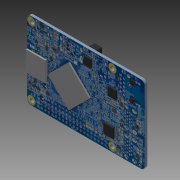
# Autodesk Inventor part: nanopi_m4_board
Saved by Autodesk Inventor 2013 SP2 (Build 170200200, 200)
## iProperties
Created: 2018-09-17
Part Number: nanopi_m4_board
Material: Generic
Document SubType Name: Modeling
Designer: alex
Density: 1 g/cm^3
Mass: 10.4345 g
Surface Area: 108.998 cm^2
Volume: 10.4345 cm^3
Author: alex
Autodesk Inventor part; units mm, degrees
ref_plane "YZ Plane" through (0, 0, 0) normal (1, 0, 0) x (0, 1, 0)
ref_plane "XZ Plane" through (0, 0, 0) normal (0, 1, 0) x (-1, 0, 0)
ref_plane "XY Plane" through (0, 0, 0) normal (0, 0, 1) x (1, 0, 0)
sketch "Sketch1" plane through (0, 0, 0) normal (0, 1, 0) x (-1, 0, 0)
  line L0 (0, 0) -> (-85, 0)
  line L1 (-85, 0) -> (-85, -56)
  line L2 (-85, -56) -> (0, -56)
  line L3 (0, -56) -> (0, 0)
  dimension "d0" = 85
  dimension "d1" = 56
  constraints: 8 end point, 2 parallel, 1 horizontal, 1 perpendicular
  measures "d0" distance of L2.end L1.end
  measures "d1" distance of L1.end L0.end
extrude "Extrusion1" add sketch "Sketch1" along normal blind 1.8
fillet "Fillet1" radius 3 4 edges at (0, 0.9, 0) (85, 0.9, 0) (85, 0.9, -56) (0, 0.9, -56)
sketch "Sketch2" plane through (0, 1.8, 0) normal (0, 1, 0) x (1, 0, 0)
  line L0 (0, 53) -> (0, 3) projected
  line L1 (3, 0) -> (82, 0) projected
  line L2 (82, 56) -> (3, 56) projected
  point P0 (0, 0)
  point P1 (3.5, 52.5)
  point P2 (61.5, 52.5)
  point P3 (3.5, 3.5)
  point P4 (61.5, 3.5)
  dimension "d5" = 58
  dimension "d7" = 49
  dimension "d8" = 3.5
  dimension "d9" = 3.5
  dimension "d10" = 3.5
  dimension "d11" = 3.5
  dimension "d12" = 3.5
  dimension "d13" = 3.5
  measures "d5" distance of point (61.5, 52.5) point (3.5, 52.5)
  measures "d7" distance of point (61.5, 3.5) point (61.5, 52.5)
  measures "d8" distance from line of L2 point (3.5, 52.5)
  measures "d9" distance from line of L0 point (3.5, 52.5)
  measures "d10" distance from line of L0 point (3.5, 3.5)
  measures "d11" distance from line of L1 point (3.5, 3.5)
  measures "d12" distance from line of L1 point (61.5, 3.5)
  measures "d13" distance from line of L2 point (61.5, 52.5)
hole "Hole1" at (3.5, 1.8, -52.5) at (61.5, 1.8, -52.5) at (3.5, 1.8, -3.5) at (61.5, 1.8, -3.5) direction (0, -1, 0) diameter 3 end through all
sketch "Sketch3" plane through (0, 0, 0) normal (0, -1, 0) x (1, 0, 0)
  line L0 (0, -53) -> (0, -3) projected
  line L1 (14.2126, -21.7399) -> (0, -21.7399)
  line L2 (0, -21.7399) -> (0, -36.2099)
  line L3 (0, -36.2099) -> (14.2126, -36.2099)
  line L4 (14.2126, -36.2099) -> (14.2126, -21.7399)
  line L5 (41.7741, -5) -> (46.9065, -5)
  line L6 (46.9065, -5) -> (46.9065, -10.2381)
  line L7 (46.9065, -10.2381) -> (41.7741, -10.2381)
  line L8 (41.7741, -10.2381) -> (41.7741, -5)
  line L9 (58.8394, -15.3064) -> (64.9983, -15.3064)
  line L10 (64.9983, -15.3064) -> (64.9983, -21.337)
  line L11 (64.9983, -21.337) -> (58.8394, -21.337)
  line L12 (58.8394, -21.337) -> (58.8394, -15.3064)
  line L13 (56.1449, -39.6854) -> (63, -39.6854)
  line L14 (63, -39.6854) -> (63, -46.55)
  line L15 (63, -46.55) -> (56.1449, -46.55)
  line L16 (56.1449, -46.55) -> (56.1449, -39.6854)
  line L17 (30.8677, -14.7931) -> (45.8159, -29.4847)
  line L18 (45.8159, -29.4847) -> (31.0297, -44.5291)
  line L19 (31.0297, -44.5291) -> (16.0816, -29.8375)
  line L20 (16.0816, -29.8375) -> (30.8677, -14.7931)
  circle A0 centre (76.4179, -4.5925) radius 1.5529
  circle A1 centre (76.4179, -15.9302) radius 1.5186
  point P0 (0, 0)
  constraints: 40 end point, 10 parallel, 5 perpendicular, 4 horizontal, 2 centre point, 1 point on line
extrude "Extrusion2" add sketch "Sketch3" along normal blind 1
sketch "Sketch4" plane through (0, 1.8, 0) normal (0, 1, 0) x (1, 0, 0)
  line L0 (6.6003, 22.2047) -> (20.4228, 22.2047)
  line L1 (20.4228, 22.2047) -> (20.4228, 10.4766)
  line L2 (20.4228, 10.4766) -> (6.6003, 10.4766)
  line L3 (6.6003, 10.4766) -> (6.6003, 22.2047)
  line L4 (44.413, 42.4767) -> (55.5812, 42.4767)
  line L5 (55.5812, 42.4767) -> (55.5812, 31.1828)
  line L6 (55.5812, 31.1828) -> (44.413, 31.1828)
  line L7 (44.413, 31.1828) -> (44.413, 42.4767)
  line L8 (44.413, 28.1626) -> (55.5812, 28.1626)
  line L9 (55.5812, 28.1626) -> (55.5812, 17.0574)
  line L10 (55.5812, 17.0574) -> (44.413, 17.0574)
  line L11 (44.413, 17.0574) -> (44.413, 28.1626)
  line L12 (57.5002, 34.8635) -> (66.4976, 34.8635)
  line L13 (66.4976, 34.8635) -> (66.4976, 25.9919)
  line L14 (66.4976, 25.9919) -> (57.5002, 25.9919)
  line L15 (57.5002, 25.9919) -> (57.5002, 34.8635)
  point P0 (0, 0)
  constraints: 32 end point, 8 parallel, 4 horizontal, 4 perpendicular
extrude "Extrusion3" add sketch "Sketch4" along normal blind 1
sketch "Sketch5" plane through (0, 1.8, 0) normal (0, 1, 0) x (1, 0, 0)
  line L0 (3.0525, 45.1901) -> (5.1263, 45.1901)
  line L1 (5.1263, 45.1901) -> (5.1263, 24.9394)
  line L2 (5.1263, 24.9394) -> (3.0525, 24.9394)
  line L3 (3.0525, 24.9394) -> (3.0525, 45.1901)
  line L4 (7.8863, 45.1901) -> (9.9602, 45.1901)
  line L5 (9.9602, 45.1901) -> (9.9602, 24.9394)
  line L6 (9.9602, 24.9394) -> (7.8863, 24.9394)
  line L7 (7.8863, 24.9394) -> (7.8863, 45.1901)
  point P0 (0, 0)
  dimension "d25" = 0
  constraints: 16 end point, 4 parallel, 2 horizontal, 2 perpendicular
  measures "d25" distance between parallel lines of L4 L0
extrude "Extrusion4" add sketch "Sketch5" along normal blind 3
sketch "Sketch6" plane through (0, 1.8, 0) normal (0, 1, 0) x (1, 0, 0)
  line L0 (41.9919, 16.3406) -> (47.3417, 16.3406)
  line L1 (47.3417, 16.3406) -> (47.3417, 0.8787)
  line L2 (47.3417, 0.8787) -> (41.9919, 0.8787)
  line L3 (41.9919, 0.8787) -> (41.9919, 16.3406)
  point P0 (0, 0)
  constraints: 8 end point, 2 parallel, 1 horizontal, 1 perpendicular
extrude "Extrusion5" add sketch "Sketch6" along normal blind 5
body "Solid1"
